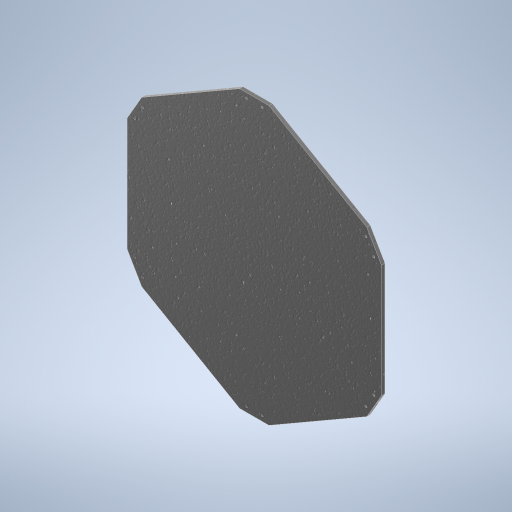
# Autodesk Inventor part: Body_Plate
Saved by Autodesk Inventor 2024 (Build 280153000, 153)
## iProperties
Created: 2024-06-03
Part Number: Body_Plate
Material: Generic
Document SubType Name: Modeling
Designer: Hemant
Density: 1 g/cm^3
Appearance: Fine Textured - Black
Author: Hemant
Autodesk Inventor part; units mm, degrees
ref_plane "YZ Plane" through (0, 0, 0) normal (1, 0, 0) x (0, 1, 0)
ref_plane "XZ Plane" through (0, 0, 0) normal (0, 1, 0) x (-1, 0, 0)
ref_plane "XY Plane" through (0, 0, 0) normal (0, 0, 1) x (1, 0, 0)
sketch "Sketch1" plane through (0, 0, 0) normal (0, 0, 1) x (1, 0, 0)
  circle A0 centre (0, 0) radius 150 construction
  line L0 (0, -150) -> (-129.9038, -75)
  line L1 (-129.9038, -75) -> (-129.9038, 75)
  line L2 (-129.9038, 75) -> (0, 150)
  line L3 (0, 150) -> (129.9038, 75)
  line L4 (129.9038, 75) -> (129.9038, -75)
  line L5 (129.9038, -75) -> (0, -150)
  circle A1 centre (0, 0) radius 6.154 construction
  line L6 (30, 0) -> (15, -25.9808) construction
  line L7 (15, -25.9808) -> (-15, -25.9808) construction
  line L8 (-15, -25.9808) -> (-30, 0) construction
  line L9 (-30, 0) -> (-15, 25.9808) construction
  line L10 (-15, 25.9808) -> (15, 25.9808) construction
  line L11 (15, 25.9808) -> (30, 0) construction
  line L12 (-129.9038, 57.6795) -> (-114.9038, 83.6603)
  line L13 (-15, 141.3397) -> (15, 141.3397)
  line L14 (129.9038, 57.6795) -> (114.9038, 83.6603)
  line L15 (129.9038, -57.6795) -> (114.9038, -83.6603)
  line L16 (-15, -141.3397) -> (15, -141.3397)
  line L17 (-129.9038, -57.6795) -> (-114.9038, -83.6603)
  line L18 (-129.9038, 75) -> (129.9038, -75) construction
  line L19 (-125.9038, 81.9282) -> (133.9038, -68.0718) construction
  line L20 (-133.9038, 68.0718) -> (125.9038, -81.9282) construction
  line L21 (-125.5737, 55.1795) -> (-110.5737, 81.1603) construction
  circle A2 centre (-114.0737, 75.0981) radius 1.1
  circle A3 centre (-122.0737, 61.2417) radius 1.1
  line L22 (-133.9038, -68.0718) -> (125.9038, 81.9282) construction
  line L23 (-129.9038, -75) -> (129.9038, 75) construction
  line L24 (-125.9038, -81.9282) -> (133.9038, 68.0718) construction
  line L25 (-110.5737, -81.1603) -> (-125.5737, -55.1795) construction
  circle A4 centre (-114.0737, -75.0981) radius 1.1
  circle A5 centre (-122.0737, -61.2417) radius 1.1
  line L26 (-8, -150) -> (-8, 150) construction
  line L27 (0, -150) -> (0, 150) construction
  line L28 (8, -150) -> (8, 150) construction
  line L29 (15, -136.3397) -> (-15, -136.3397) construction
  circle A6 centre (8, -136.3397) radius 1.1
  circle A7 centre (-8, -136.3397) radius 1.1
  line L30 (125.9038, -81.9282) -> (-133.9038, 68.0718) construction
  line L31 (129.9038, -75) -> (-129.9038, 75) construction
  line L32 (133.9038, -68.0718) -> (-125.9038, 81.9282) construction
  line L33 (125.5737, -55.1795) -> (110.5737, -81.1603) construction
  circle A8 centre (122.0737, -61.2417) radius 1.1
  circle A9 centre (114.0737, -75.0981) radius 1.1
  line L34 (133.9038, 68.0718) -> (-125.9038, -81.9282) construction
  line L35 (129.9038, 75) -> (-129.9038, -75) construction
  line L36 (125.9038, 81.9282) -> (-133.9038, -68.0718) construction
  line L37 (110.5737, 81.1603) -> (125.5737, 55.1795) construction
  circle A10 centre (114.0737, 75.0981) radius 1.1
  circle A11 centre (122.0737, 61.2417) radius 1.1
  line L38 (8, 150) -> (8, -150) construction
  line L39 (0, 150) -> (0, -150) construction
  line L40 (-8, 150) -> (-8, -150) construction
  line L41 (-15, 136.3397) -> (15, 136.3397) construction
  circle A12 centre (-8, 136.3397) radius 1.1
  circle A13 centre (8, 136.3397) radius 1.1
  dimension "d5" = 300
  dimension "d6" = 30
  dimension "d7" = 30
  dimension "d8" = 30
  dimension "d9" = 30
  dimension "d10" = 30
  dimension "d11" = 30
  dimension "d12" = 30
  dimension "d17" = 8
  dimension "d18" = 8
  dimension "d19" = 5
  dimension "d20" = 2.2
  dimension "d21" = 2.2
  dimension "d24" = 360
  constraints: 84 end point, 36 point on line, 13 centre point, 8 parallel, 3 coincident, 2 vertical alignment, 1 horizontal, 1 horizontal alignment, 1 perpendicular, 127 other
  measures "d6" distance of L9.end L10.end
  measures "d7" distance of L13.start L13.end
  measures "d8" distance of L12.start L12.end
  measures "d9" distance of L17.start L17.end
  measures "d10" distance of L15.start L15.end
  measures "d11" distance of L14.start L14.end
  measures "d12" distance of L16.start L16.end
  measures "d17" distance between parallel lines of L18 L19
  measures "d18" distance between parallel lines of L18 L20
  measures "d19" distance between parallel lines of L12 L21
  measures "d20" diameter of A2
  measures "d21" diameter of A3
extrude "Extrusion1" add sketch "Sketch1" along normal blind 3.5 contours L0 L17 L1 L12 L2 L13 L3 L14 L4 L15 L5 L16
body "Solid1"
